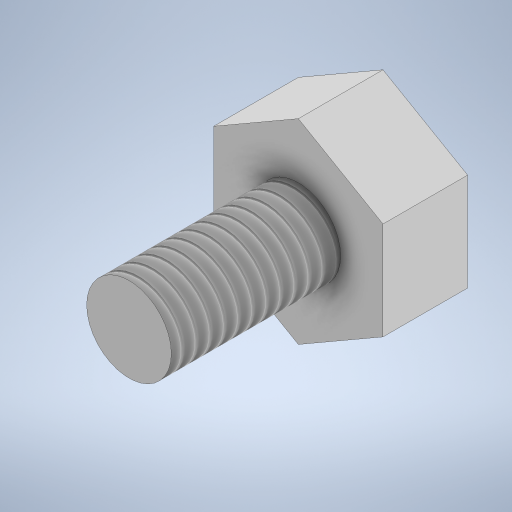
# Autodesk Inventor part: m3 bolt long
Saved by Autodesk Inventor 2023 (Build 270158000, 158)
## iProperties
Created: 2023-06-05
Part Number: m3 bolt long
Material: Generic
Document SubType Name: Modeling
Designer: Ronan
Density: 1 g/cm^3
Appearance: Default
Author: Ronan
Autodesk Inventor part; units mm, degrees
ref_plane "YZ Plane" through (0, 0, 0) normal (1, 0, 0) x (0, 1, 0)
ref_plane "XZ Plane" through (0, 0, 0) normal (0, 1, 0) x (-1, 0, 0)
ref_plane "XY Plane" through (0, 0, 0) normal (0, 0, 1) x (1, 0, 0)
sketch "Sketch1" plane through (0, 0, 0) normal (0, 0, 1) x (1, 0, 0)
  line L0 (3, 1.7321) -> (3, -1.7321)
  line L1 (3, 1.7321) -> (0, 3.4641)
  line L2 (-3, 1.7321) -> (0, 3.4641)
  line L3 (0, -3.4641) -> (3, -1.7321)
  line L4 (-3, 1.7321) -> (-3, -1.7321)
  line L5 (-3, -1.7321) -> (0, -3.4641)
  point P0 (0, 0)
  point P1 (0, 0)
  point P2 (0, 0)
  point P3 (0, 0)
  point P4 (0, 0)
  point P5 (0, 0)
  dimension "d0" = 120
  dimension "d1" = 120
  dimension "d2" = 120
  dimension "d3" = 120
  dimension "d4" = 120
  dimension "d5" = 120
  dimension "d6" = 6
  dimension "d7" = 3
  dimension "d18" = 0
  dimension "d19" = 0
  dimension "d20" = 0
  constraints: 12 end point, 3 coincident, 2 vertical
  measures "d0" angle of L3 L0
  measures "d1" angle of L5 L3
  measures "d2" angle of L5 L4
  measures "d3" angle of L4 L2
  measures "d4" angle of L2 L1
  measures "d5" angle of L1 L0
  measures "d6" distance between parallel lines of L0 L4
  measures "d7" distance from line of L4 point (0, 0)
  measures "d18" distance of point (0, 0) point (0, 0)
  measures "d19" horizontal distance of L1.end point (0, 0)
  measures "d20" horizontal distance of point (0, 0) L3.start
extrude "Extrusion1" add sketch "Sketch1" along normal blind 3
sketch "Sketch2" plane through (0, 0, 3) normal (0, 0, 1) x (1, 0, 0)
  circle A0 centre (0, 0) radius 1.5
  dimension "d10" = 3
  constraints: 1 centre point, 1 coincident
  measures "d10" diameter of A0
extrude "Extrusion2" add sketch "Sketch2" along normal blind 6
thread "Thread2" size "M3x0.5" class "6g" standard "ANSI Metric M Profile" full length
body "Solid1"
